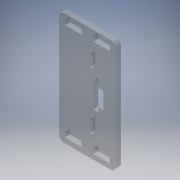
# Autodesk Inventor part: Front_wall
Saved by Autodesk Inventor 2016 (Build 200138000, 138)
## iProperties
Created: 2015-06-25
Part Number: Front_wall
Material: Generic
Document SubType Name: Modeling
Designer: Openlab
Density: 1 g/cm^3
Appearance: Polycarbonate - Clear
Author: Openlab
Autodesk Inventor part; units mm, degrees
ref_plane "YZ Plane" through (0, 0, 0) normal (1, 0, 0) x (0, 1, 0)
ref_plane "XZ Plane" through (0, 0, 0) normal (0, 1, 0) x (-1, 0, 0)
ref_plane "XY Plane" through (0, 0, 0) normal (0, 0, 1) x (1, 0, 0)
sketch "Sketch1" plane through (0, 0, 0) normal (0, 1, 0) x (-1, 0, 0)
  line L0 (17, -20.2435) -> (17, -42.6397) construction
  line L1 (13.2323, -33.5) -> (6.4845, -33.5) construction
  line L2 (34, -64) -> (34, -3)
  line L3 (0, -3) -> (0, -64)
  line L4 (31, 0) -> (3, 0)
  line L5 (3, -67) -> (31, -67)
  line L6 (15.3, -20) -> (13.5, -20)
  line L7 (13.5, -20) -> (13.5, -13)
  line L8 (13.5, -13) -> (15.3, -13)
  line L9 (15.3, -13) -> (15.3, -20)
  line L10 (30.5, -3) -> (20.5, -3)
  line L11 (20.5, -3) -> (20.5, -6)
  line L12 (20.5, -6) -> (30.5, -6)
  line L13 (30.5, -6) -> (30.5, -3)
  line L14 (13.5, -3) -> (3.5, -3)
  line L15 (3.5, -3) -> (3.5, -6)
  line L16 (3.5, -6) -> (13.5, -6)
  line L17 (13.5, -6) -> (13.5, -3)
  line L18 (30.5, -61) -> (20.5, -61)
  line L19 (20.5, -61) -> (20.5, -64)
  line L20 (20.5, -64) -> (30.5, -64)
  line L21 (30.5, -64) -> (30.5, -61)
  line L22 (13.5, -61) -> (3.5, -61)
  line L23 (3.5, -61) -> (3.5, -64)
  line L24 (3.5, -64) -> (13.5, -64)
  line L25 (13.5, -64) -> (13.5, -61)
  line L26 (10.5, -28.5) -> (7.5, -28.5)
  line L27 (7.5, -28.5) -> (7.5, -38.5)
  line L28 (7.5, -38.5) -> (10.5, -38.5)
  line L29 (10.5, -28.5) -> (10.5, -26)
  line L30 (10.5, -26) -> (13.5, -26)
  line L31 (13.5, -26) -> (13.5, -41)
  line L32 (13.5, -41) -> (10.5, -41)
  line L33 (10.5, -41) -> (10.5, -38.5)
  arc A0 (34, -3) -> (31, 0) centre (31, -3) ccw
  arc A1 (31, -67) -> (34, -64) centre (31, -64) ccw
  arc A2 (0, -64) -> (3, -67) centre (3, -64) ccw
  arc A3 (3, 0) -> (0, -3) centre (3, -3) ccw
  line L34 (15.3, -47) -> (13.5, -47)
  line L35 (13.5, -47) -> (13.5, -54)
  line L36 (13.5, -54) -> (15.3, -54)
  line L37 (15.3, -54) -> (15.3, -47)
  point P0 (0, 0)
  dimension "d22" = 7
  dimension "d24" = 1.8
  dimension "d27" = 10
  dimension "d28" = 3
  dimension "d30" = 3
  dimension "d31" = 7
  dimension "d33" = 10
  dimension "d34" = 15
  dimension "d35" = 6
  dimension "d37" = 67
  dimension "d39" = 7
  dimension "d44" = 3.5
  dimension "d48" = 3.5
  dimension "d50" = 20.5
  constraints: 76 end point, 15 parallel, 12 perpendicular, 10 point on line, 9 horizontal, 8 point on circle, 8 tangent, 7 equal length, 4 centre point, 3 equal radius, 2 collinear, 2 vertical, 6 other
  measures "d22" distance of L8.end L6.start
  measures "d24" distance of L7.end L8.end
  measures "d27" distance of L11.end L12.end
  measures "d28" distance of L14.end L15.end
  measures "d30" distance between parallel lines of L5 L24
  measures "d31" distance between parallel lines of L17 L11
  measures "d33" distance of L26.end L27.end
  measures "d34" distance of L30.end L31.end
  measures "d35" diameter of A0
  measures "d37" distance between parallel lines of L5 L4
  measures "d39" distance between parallel lines of L8 L12
  measures "d44" distance between parallel lines of L13 L2
  measures "d48" distance between parallel lines of L3 L15
  measures "d50" distance between parallel lines of L31 L2
extrude "Extrusion1" add sketch "Sketch1" along normal blind 3
body "Solid1"
